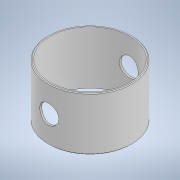
# Autodesk Inventor part: 75. Втулка шестерни второй передачи
Saved by Autodesk Inventor 2021 (Build 250183000, 183)
## iProperties
Created: 2021-03-15
Part Number: 75. Втулка шестерни второй передачи
Material: Типовые
Document SubType Name: Modeling
Designer: Данил
Density: 1 g/cm^3
Appearance: По умолчанию
Author: Данил
Autodesk Inventor part; units mm, degrees
ref_plane "YZ Plane" through (0, 0, 0) normal (1, 0, 0) x (0, 1, 0)
ref_plane "XZ Plane" through (0, 0, 0) normal (0, 1, 0) x (-1, 0, 0)
ref_plane "XY Plane" through (0, 0, 0) normal (0, 0, 1) x (1, 0, 0)
sketch "Эскиз1" plane through (0, 0, 0) normal (0, 0, 1) x (1, 0, 0)
  line L0 (0, 14) -> (0, -14)
  line L1 (21, 14) -> (21.6, 14)
  line L2 (22, 13.6) -> (22, -13.6)
  line L3 (21.6, -14) -> (21, -14)
  line L4 (21, -14) -> (21, 14)
  line L5 (22, 13.6) -> (21.6, 14)
  line L6 (22, -13.6) -> (21.6, -14)
  point P0 (0, 0)
  point P1 (0, 0)
  point P2 (22, -14)
  point P3 (22, 14)
  dimension "d0" = 28
  dimension "d1" = 44
  dimension "d2" = 42
  dimension "d3" = 0.4
  dimension "d4" = 45
  dimension "d5" = 0.4
  dimension "d6" = 45
  constraints: 14 end point, 4 point on line, 2 horizontal alignment, 2 parallel, 1 coincident, 1 horizontal, 1 midpoint, 1 perpendicular, 1 vertical
  measures "d0" distance of L0.start L0.end
  measures "d1" diameter of L2 L0
  measures "d2" diameter of L4 L0
  measures "d3" distance of L2.start point (22, 14)
  measures "d4" angle of L2 L5
  measures "d5" distance of L2.end point (22, -14)
  measures "d6" angle of L2 L6
revolve "Вращение1" add sketch "Эскиз1" angle 360 about axis through (0, 14, 0) along (0, -1, 0)
sketch "Эскиз2" plane through (0, 0, 0) normal (0, 0, 1) x (1, 0, 0)
  circle A0 centre (0, 0) radius 5
  dimension "d8" = 10
  constraints: 1 centre point, 1 coincident
  measures "d8" diameter of A0
extrude "Выдавливание1" cut sketch "Эскиз2" along normal through all both and the other way through all
equation "\"d5\" = d3"
equation "\"d6\" = d4"
